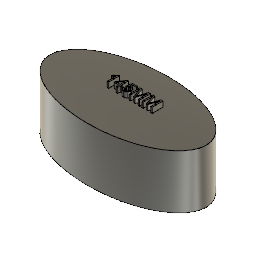
STLExampleWidget (Autodesk Fusion 360 design; units mm, degrees)
Autodesk Fusion 360 part; units mm, degrees
sketch "Object" plane through (0, 0, 0) normal (0, 0, 1) x (1, 0, 0)
  ellipse E0 centre (0, 0) end of major axis (-72.5, 0) minor radius 37.5
  line L0 (72.5, 0) -> (-72.5, 0)
  line L1 (0, 37.5) -> (0, -37.5)
  dimension "d3" = 145
  dimension "d4" = 75
  constraint coincident E0 L0.start
  constraint coincident E0 L0.end
  constraint coincident E0 L1.start
  constraint coincident E0 L1.end
  constraint coincident E0.centre origin
  constraint horizontal L0
  measures "d3" distance of E0
extrude "Extrude1" add sketch "Object" along normal blind 50
sketch "Text" plane through (0, 0, 50) normal (0, 0, 1) x (-1, 0, 0)
  ellipse E0 centre (0, 0) end of major axis (72.5, 0) minor radius 37.5
  line L0 (28.8798, 10.4043) -> (-28.8798, 10.4043) construction
  line L1 (-28.8798, 10.4043) -> (-28.8798, -10.4043) construction
  line L2 (-28.8798, -10.4043) -> (28.8798, -10.4043) construction
  line L3 (28.8798, -10.4043) -> (28.8798, 10.4043) construction
  line L4 (0, -55.4268) -> (0, 66.777) construction
  line L5 (70.5204, 0) -> (-72.8231, 0) construction
  dimension "d7" = 10
  text T0 "145MM" font "Arial" height 10 align centre top in box 57.7595 x 20.8087 at (28.8798, 10.4043) x (-1, 0) y (0, -1) spacing 1
  constraint vertical L4
  constraint coincident E0.centre L4
  constraint coincident L4
  constraint perpendicular L4 L5
  constraint coincident E0.centre L5
  constraint coincident L5
emboss "Emboss1" depth 5 profiles "Text" section 1 text T0 onto face at (-13.6816, 12.1083, 50)
equation "d3 = majorAxis"
equation "majorAxis = 145.0 mm"
